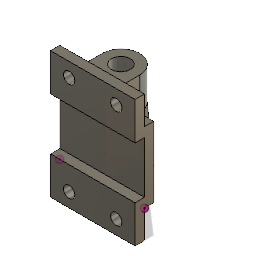
QWEwwe (4) (Autodesk Fusion 360 design; units mm, degrees)
Autodesk Fusion 360 part; units mm, degrees
sketch "Sketch1" plane through (0, 0, 0) normal (0, 1, 0) x (1, 0, 0)
  line L0 (-90, 0) -> (0, 0)
  line L1 (0, 0) -> (0, -10)
  line L2 (0, -10) -> (-90, -10)
  line L3 (-90, -10) -> (-90, 0)
  line L4 (-90, 0) -> (-90, 45)
  arc A0 (-50, 45) -> (-90, 45) centre (-70, 45) ccw
  line L5 (-50, 45) -> (-50, 10)
  line L6 (-50, 10) -> (0, 10)
  line L7 (0, 10) -> (0, -3.1399)
  dimension "d1" = 10
  dimension "d2" = 45
  dimension "d3" = 40
  constraint coincident L0.end L1.start
  constraint horizontal L0
  constraint perpendicular L0 L1
  constraint perpendicular L1 L2
  constraint perpendicular L0 L3
  constraint perpendicular L0 L4
  constraint perpendicular L0 L5
  constraint perpendicular L5 L6
  constraint coincident L1 L7.end
  constraint perpendicular L0 L7
  measures "d1" distance of L0.end L1.end
  measures "d2" distance of L0.start L4.end
  measures "d3" distance of L4.end A0.start
extrude "Extrude1" add sketch "Sketch1" along normal blind 75 contours L0 L4 A0 L5 L6 L7
sketch "Sketch2" plane through (0, 0, 0) normal (0, 1, 0) x (1, 0, 0)
  point P0 (-90, 0)
sketch "Sketch3" plane through (0, 0, 0) normal (0, 1, 0) x (1, 0, 0)
  line L0 (-90, -10) -> (-90, 0)
  line L1 (0, 0) -> (-90, 0)
  line L2 (-90, -10) -> (0, -10)
  line L3 (0, -10) -> (0, 0)
  point P0 (-90, 0)
  point P1 (0, -10)
  constraint coincident L1.start L3.end
  constraint coincident P0 L0.end
  constraint coincident L0.start L2.start
  constraint coincident P1 L2.end
extrude "Extrude2" add sketch "Sketch3" along normal blind 105
sketch "Sketch4" plane through (0, 0, 10) normal (0, 0, 1) x (1, 0, 0)
  line L0 (-90, 0) -> (0, 0)
  line L1 (0, 0) -> (0, 105)
  line L2 (0, 105) -> (-90, 105)
  line L3 (-90, 105) -> (-90, 0)
  line L4 (0, 0) -> (-90, 0)
  line L5 (-90, 0) -> (-90, -30)
  line L6 (-90, -30) -> (0, -30)
  line L7 (0, -30) -> (0, 0)
  dimension "d9" = 30
  constraint coincident L0.end L1.start
  constraint coincident L0.start L3.end
  constraint perpendicular L4 L5
  constraint perpendicular L5 L6
  constraint perpendicular L4 L7
  measures "d9" distance of L0.start L5.end
extrude "Extrude3" add sketch "Sketch4" against normal blind 10 contours L0 L4 L5 L6 L7
sketch "Sketch5" plane through (0, 0, 0) normal (1, 0, 0) x (0, 0, -1)
  line L0 (0, 0) -> (10, 0)
  line L1 (10, 0) -> (10, 75)
  line L2 (10, 75) -> (0, 75)
  line L3 (0, 75) -> (0, 105)
  line L4 (0, 105) -> (-10, 105)
  line L5 (-10, 105) -> (-10, -30)
  line L6 (-10, -30) -> (0, -30)
  line L7 (0, -30) -> (0, 0)
  line L8 (0, 65) -> (-10, 65)
  line L9 (0, 65) -> (0, 10)
  line L10 (-10, 10) -> (-10, 65)
  line L11 (-10, 65) -> (-10, 10)
  line L12 (-10, 10) -> (0, 10)
  dimension "d12" = 10
  dimension "d13" = 10
  constraint coincident L5 L8.end
  constraint perpendicular L8 L9
  constraint coincident L5 L10.start
  constraint perpendicular L8 L10
  measures "d12" distance of L2.end L8.start
  measures "d13" distance of L0.start L9.end
extrude "Extrude4" cut sketch "Sketch5" against normal blind 135 contours L5 L8 L9 L10 L11 L12
sketch "Sketch6" plane through (0, 75, 0) normal (0, 1, 0) x (-1, 0, 0)
  arc A0 (50, -45) -> (90, -45) centre (70, -45) ccw
  line L0 (90, -45) -> (90, 0)
  line L1 (90, 0) -> (0, 0)
  line L2 (0, 0) -> (0, -10)
  line L3 (0, -10) -> (50, -10)
  line L4 (50, -10) -> (50, -45)
  circle A1 centre (70, -45) radius 10
  dimension "d16" = 20
  constraint concentric A0 A1
  measures "d16" diameter of A1
extrude "Extrude5" cut sketch "Sketch6" against normal blind 95 contours A1
sketch "Sketch7" plane through (0, 0, 0) normal (0, 0, -1) x (-1, 0, 0)
sketch "Sketch8" plane through (0, 0, 0) normal (0, 0, -1) x (-1, 0, 0)
  line L0 (0, 75) -> (90, 75)
  line L1 (90, 75) -> (90, 105)
  line L2 (90, 105) -> (0, 105)
  line L3 (0, 105) -> (0, 75)
  circle A0 centre (20, 90) radius 6
  circle A1 centre (70, 90) radius 6
  line L4 (0, -30) -> (90, -30)
  circle A2 centre (70, -15) radius 6
  circle A3 centre (20, -15) radius 6
  dimension "d20" = 12
  dimension "d21" = 50
  dimension "d22" = 12
  dimension "d24" = 12
  dimension "d26" = 12
  measures "d20" diameter of A0
  measures "d21" distance of A0.centre A1.centre
  measures "d22" diameter of A1
  measures "d24" diameter of A2
  measures "d26" diameter of A3
extrude "Extrude6" cut sketch "Sketch8" against normal blind 30 contours A0 | A1 | A2 | A3
sketch "Sketch9" plane through (0, 0, 0) normal (0, 0, -1) x (-1, 0, 0)
  circle A0 centre (20, 90) radius 6
  circle A1 centre (70, 90) radius 6
  line L0 (0, 75) -> (90, 75)
  line L1 (90, 75) -> (90, 105)
  line L2 (90, 105) -> (0, 105)
  line L3 (0, 105) -> (0, 75)
  line L4 (0, 105) -> (37, 105)
  line L5 (37, 105) -> (37, 75)
  line L6 (37, 105) -> (43, 105)
  line L7 (43, 105) -> (43, 75)
  line L8 (37, 75) -> (43, 75)
  dimension "d29" = 37
  dimension "d30" = 6
  constraint coincident L2.end L3.start
  constraint perpendicular L3 L4
  constraint coincident L0 L5.end
  constraint perpendicular L5 L6
  constraint coincident L0 L7.end
  measures "d29" distance of L2.end L4.end
  measures "d30" distance of L4.end L6.end
extrude "Extrude7" add sketch "Sketch9" along normal blind 10 contours L0 L2 L5 L6 L7 L8
chamfer "Chamfer1" distance 30 distance2 10 1 edges at (-40, 105, -10) measured on face at (-29, 25, -10)
sketch "Sketch10" plane through (0, 0, 0) normal (0, 0, -1) x (-1, 0, 0)
  circle A0 centre (20, -15) radius 6
  circle A1 centre (70, -15) radius 6
  line L0 (0, 0) -> (0, -30)
  line L1 (0, -30) -> (90, -30)
  line L2 (90, -30) -> (90, 0)
  line L3 (90, 0) -> (0, 0)
  line L4 (0, -30) -> (37, -30)
  line L5 (37, -30) -> (37, 0)
  line L6 (37, 0) -> (43, 0)
  line L7 (43, 0) -> (43, -30)
  line L8 (37, -30) -> (43, -30)
  dimension "d35" = 37
  dimension "d36" = 6
  constraint coincident L0.end L1.start
  constraint perpendicular L0 L4
  constraint vertical L5
  constraint coincident L3 L5.end
  constraint perpendicular L5 L6
  constraint coincident L1 L7.end
  measures "d35" distance of L0.end L4.end
  measures "d36" distance of L5.end L6.end
extrude "Extrude8" add sketch "Sketch10" along normal blind 10 contours L1 L3 L5 L6 L7 L8
chamfer "Chamfer2" distance 30 distance2 10 1 edges at (-40, -30, -10) measured on face at (-24.6201, 25, -10)
sketch "Sketch11" plane through (-50, 0, 0) normal (1, 0, 0) x (0, 0, -1)
  line L0 (10, 0) -> (45, 0)
  line L1 (45, 0) -> (45, 75)
  line L2 (45, 75) -> (10, 75)
  line L3 (10, 75) -> (10, 0)
sketch "Sketch12" plane through (0, 0, 0) normal (1, 0, 0) x (0, 0, -1)
  line L0 (0, 10) -> (-10, 10)
  line L1 (-10, 10) -> (-10, -30)
  line L2 (-10, -30) -> (0, -30)
  line L3 (0, -30) -> (0, 0)
  line L4 (0, 0) -> (10, 0)
  line L5 (10, 0) -> (10, 75)
  line L6 (10, 75) -> (0, 75)
  line L7 (0, 75) -> (0, 105)
  line L8 (0, 105) -> (-10, 105)
  line L9 (-10, 105) -> (-10, 65)
  line L10 (-10, 65) -> (0, 65)
  line L11 (0, 65) -> (0, 10)
ref_plane "WorkPlane1" through (0, 37.5, 0) normal (0, 1, 0) x (0, 0, 1)
sketch "Sketch13" plane through (0, 37.5, 0) normal (0, 1, 0) x (1, 0, 0)
  arc A0 (-50, 45) -> (-90, 45) centre (-70, 45) ccw
  line L0 (0, 10) -> (-54.3666, 57.4739)
  point P0 (0, 10)
  constraint coincident P0 L0.start
  constraint coincident A0 L0.end
rib "Rib1" add thickness 6 on both sides direction (-0.657744, 0, 0.753242) up to next extending the curves path "Sketch13" along L0
fillet "Fillet1" radius 152.5 1 edges at (-54.3666, 37.5, -57.4739)
